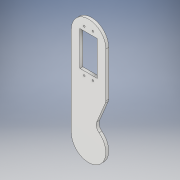
# Autodesk Inventor part: Pata - Brazo
Saved by Autodesk Inventor 2019 (Build 230136000, 136)
## iProperties
Created: 2020-02-12
Part Number: Pata - Brazo
Material: ABS Plastic
Document SubType Name: Modeling
Designer: jacqu
Density: 1.06 g/cm^3
Appearance: Smooth - White
Mass: 6.41843 g
Surface Area: 58.6028 cm^2
Volume: 6.05512 cm^3
Author: jacqu
Autodesk Inventor part; units mm, degrees
ref_plane "YZ Plane" through (0, 0, 0) normal (1, 0, 0) x (0, 1, 0)
ref_plane "XZ Plane" through (0, 0, 0) normal (0, 1, 0) x (-1, 0, 0)
ref_plane "XY Plane" through (0, 0, 0) normal (0, 0, 1) x (1, 0, 0)
sketch "Sketch1" plane through (0, 0, 0) normal (0, 0, 1) x (1, 0, 0)
  arc A0 (20, 0) -> (-20, 0) centre (0, 0) ccw
  line L0 (-20, 0) -> (-20, -104)
  line L1 (20, 0) -> (20, -52)
  arc A1 (19.4895, -54.5451) -> (20, -52) centre (13.4, -52) ccw
  arc A2 (-20, -104) -> (-7.0525, -122.7153) centre (0, -104) ccw
  arc A3 (-7.0525, -122.7153) -> (19.963, -105.2168) centre (0, -104) ccw
  arc A4 (19.963, -105.2168) -> (12.0286, -88.0215) centre (0, -104) ccw
  arc A5 (9.4588, -78.5451) -> (12.0286, -88.0215) centre (16.84, -81.6301) ccw
  line L2 (9.4588, -78.5451) -> (19.4895, -54.5451)
  line L3 (-10, 5.5) -> (10, 5.5)
  line L4 (10, 5.5) -> (10, -34.5)
  line L5 (10, -34.5) -> (-10, -34.5)
  line L6 (-10, -34.5) -> (-10, 5.5)
  dimension "d3" = 20
  dimension "d5" = 52
  dimension "d6" = 20
  dimension "d7" = 20
  dimension "d8" = 8
  dimension "d10" = 6.6
  dimension "d11" = 24
  dimension "d17" = 20
  dimension "d18" = 40
  dimension "d19" = 10
  dimension "d20" = 104
  dimension "d30" = 5.5
  constraints: 14 end point, 13 point on circle, 8 tangent, 6 centre point, 3 parallel, 1 coincident, 1 concentric, 1 horizontal, 1 perpendicular, 1 vertical alignment
  measures "d3" radius of A0
  measures "d5" distance of L1.start L1.end
  measures "d6" radius of A2
  measures "d7" radius of A4
  measures "d8" radius of A5
  measures "d10" radius of A1
  measures "d11" vertical distance of L2.start L2.end
  measures "d17" distance of L3.start L3.end
  measures "d18" distance of L3.end L4.end
  measures "d19" distance from line of L6 point (0, 0)
  measures "d20" distance of L0.start L0.end
  measures "d30" distance from line of point (0, 0) L3
extrude "Extrusion1" add sketch "Sketch1" along normal blind 3.3
sketch "Sketch2" plane through (0, 0, 3.3) normal (0, 0, 1) x (1, 0, 0)
  line L0 (-10, 5.5) -> (10, 5.5) projected
  line L1 (10, -34.5) -> (-10, -34.5) projected
  circle A0 centre (-5, 10.25) radius 1
  circle A1 centre (-5, -39.25) radius 1
  line L2 (-10, -34.5) -> (-10, 5.5) projected
  line L3 (10, 5.5) -> (10, -34.5) projected
  circle A2 centre (5, 10.25) radius 1
  circle A3 centre (5, -39.25) radius 1
  point P0 (0, 0)
  dimension "d31" = 2
  dimension "d32" = 2
  dimension "d34" = 4.75
  dimension "d36" = 4.75
  dimension "d65" = 5
  dimension "d66" = 10
  dimension "d67" = 5
  dimension "d68" = 10
  constraints: 4 centre point, 2 equal radius, 2 horizontal alignment
  measures "d31" diameter of A0
  measures "d32" diameter of A1
  measures "d34" distance from line of L0 A0.centre
  measures "d36" distance from line of L1 A1.centre
  measures "d65" distance from line of A0.centre L2
  measures "d66" distance of A0.centre A2.centre
  measures "d67" distance from line of L2 A1.centre
  measures "d68" distance of A3.centre A1.centre
extrude "Extrusion2" cut sketch "Sketch2" against normal blind 4.75 contours A0 | A1 | A2 | A3
sketch "Sketch3" plane through (0, 0, 3.3) normal (0, 0, 1) x (1, 0, 0)
  line L0 (-20, 0) -> (-20, -104) projected
  line L1 (10, 5.5) -> (10, -34.5) projected
  line L2 (10, -34.5) -> (-10, -34.5) projected
  line L3 (-10, -34.5) -> (-10, 5.5) projected
  line L4 (-10, 5.5) -> (10, 5.5) projected
  line L5 (-20, 0) -> (-20, -104) projected
  arc A0 (-20, -104) -> (12.0286, -88.0215) centre (0, -104) ccw projected
  arc A1 (9.4588, -78.5451) -> (12.0286, -88.0215) centre (16.84, -81.6301) ccw projected
  line L6 (9.4588, -78.5451) -> (19.4895, -54.5451) projected
  arc A2 (19.4895, -54.5451) -> (20, -52) centre (13.4, -52) ccw projected
  line L7 (20, -52) -> (20, 0) projected
  arc A3 (20, 0) -> (-20, 0) centre (0, 0) ccw projected
  line L8 (-15, -86) -> (-15, -56)
  line L9 (15, -45.2979) -> (15, -53.2979)
  line L10 (15, -53.2979) -> (4.448, -78.5451)
  line L11 (4.448, -78.5451) -> (-15, -86)
  line L12 (9.4588, -78.5451) -> (19.4895, -54.5451) projected
  line L13 (-15, -94.5676) -> (-15, -104)
  arc A4 (-15, -104) -> (9.0215, -92.0161) centre (0, -104) ccw
  arc A5 (-20, -104) -> (12.0286, -88.0215) centre (0, -104) ccw projected
  arc A6 (4.9629, -86.9153) -> (9.0215, -92.0161) centre (16.84, -81.6301) ccw
  arc A7 (9.4588, -78.5451) -> (12.0286, -88.0215) centre (16.84, -81.6301) ccw projected
  line L14 (4.9629, -86.9153) -> (-15, -94.5676)
  line L15 (-15, -56) -> (15, -45.2979)
  line L16 (-15, -50.6914) -> (15, -39.9893)
  line L17 (15, -39.9893) -> (15, -36.8041)
  line L18 (15, -36.8041) -> (-15, -47.5062)
  line L19 (-15, -47.5062) -> (-15, -50.6914)
  point P0 (19.8711, -53.2979)
  dimension "d45" = 5
  dimension "d46" = 5
  dimension "d48" = 8
  dimension "d49" = 18
  dimension "d52" = 5
  dimension "d54" = 3
  dimension "d56" = 30
  dimension "d57" = 8
  constraints: 22 end point, 6 parallel, 5 point on circle, 3 vertical, 3 vertical alignment, 2 centre point, 2 concentric, 2 horizontal alignment, 2 tangent
  measures "d45" distance between parallel lines of L8 L0
  measures "d46" distance between parallel lines of L7 L9
  measures "d48" distance from line of L8.start L14
  measures "d49" vertical distance of L0.end L8.start
  measures "d52" distance between parallel lines of L15 L16
  measures "d54" distance between parallel lines of L16 L18
  measures "d56" distance of L8.start L8.end
  measures "d57" distance of L9.start L9.end
equation "\"d3\" = radio_muslo"
equation "\"d6\" = radio_muslo"
equation "\"d7\" = d6"
equation "\"d17\" = base_servo"
equation "\"d18\" = altura_servo"
equation "\"d19\" = 0.5 * base_servo"
equation "\"d20\" = 2 * d5"
equation "\"d22\" = espesor"
equation "\"d31\" = agujero_servo"
equation "\"d32\" = agujero_servo"
equation "\"d34\" = distancia_agujero_servo"
equation "\"d36\" = distancia_agujero_servo"
equation "\"espesor\" = 3.3"
equation "\"radio_muslo\" = 20"
equation "\"base_servo\" = 20"
equation "\"altura_servo\" = 40"
equation "\"agujero_servo\" = 2"
equation "\"distancia_agujero_servo\" = 4.75"
body "Solid1"
